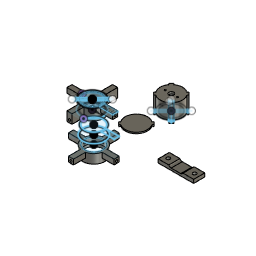
TurnstileAntenna (Autodesk Fusion 360 design; units mm, degrees)
Autodesk Fusion 360 part; units mm, degrees
note: some values were not read from the file. Set by a fixed rule: which face or edge a step refers to.
sketch "Sketch1" plane through (0, 0, 0) normal (0, 0, 1) x (1, 0, 0) in component "BOTTOM"
  circle A0 centre (0, 0) radius 20.15
  circle A1 centre (0, 0) radius 22
  dimension "d1" = 40.3
  constraint coincident A0.centre A1.centre
  measures "d1" diameter of A0
extrude "Extrude1" add sketch "Sketch1" along normal blind 17 and the other way blind 4 makes body 1 in component "BOTTOM"
sketch "Sketch1 (1)" plane through (0, 0, 17) normal (0, 0, 1) x (-1, 0, 0) in component "BOTTOM"
  circle A0 centre (0, 0) radius 20.15
  circle A1 centre (0, 0) radius 22
  circle A2 centre (0, 0) radius 20.15
  circle A3 centre (0, 0) radius 18
  point P0 (20.15, 0)
  constraint coincident A0.centre A1.centre
  constraint coincident A2 P0
extrude "Extrude2" add sketch "Sketch1 (1)" against normal blind 15 contours A0 A2 bodies 1 in component "BOTTOM"
sketch "Sketch2" plane through (0, 0, 17) normal (0, 0, 1) x (-1, 0, 0) in component "BOTTOM"
  line L0 (-20, 5) -> (-45, 5)
  line L1 (-45, 5) -> (-45, -5)
  line L2 (-45, -5) -> (-20, -5)
  line L3 (-20, -5) -> (-20, 5)
  dimension "d11" = 25
  dimension "d12" = 10
  constraint horizontal L0
  constraint vertical L1
  constraint horizontal L2
  constraint vertical L3
  measures "d11" distance of L0.start L0.end
  measures "d12" distance of L0.start L2.end
extrude "Extrude3" add sketch "Sketch2" along normal blind -9 and the other way blind 0 bodies 1 in component "BOTTOM"
pattern_circular "C-Pattern1" count 4 over 360 about axis through (0, 0, 1.75) along (0, 0, 1) of "Extrude3" in component "BOTTOM"
hole "Hole1" at (45, 0, 12.5) direction (-1, 0, 0) diameter 4.4 depth 99 tip angle 180 bodies 1 in component "BOTTOM"
extrude "Extrude4" add sketch "Sketch1 (1)" along normal blind -1 and the other way blind -1 contours A3 bodies 1 in component "BOTTOM"
extrude "Extrude5" add 1 faces at (1.6667, -29.2829, 17) along direction (0, 0, 1) blind 1 on bodies 1 bodies 1 in component "BOTTOM"
sketch "Sketch1 (2)" plane through (0, 0, 0) normal (0, 0, 1) x (1, 0, 0) in component "UPPER"
  circle A0 centre (0, 0) radius 20.1
  circle A1 centre (0, 0) radius 22
  dimension "d1_1" = 40.2
  constraint coincident A0.centre A1.centre
  measures "d1_1" diameter of A0
extrude "Extrude1'" add sketch "Sketch1 (2)" along normal blind 17 separate body makes body 2 in component "UPPER"
sketch "Sketch1 (1) (2)" plane through (0, 0, 17) normal (0, 0, 1) x (-1, 0, 0) in component "UPPER"
  circle A0 centre (0, 0) radius 20.1
  circle A1 centre (0, 0) radius 22
  circle A2 centre (0, 0) radius 20.1
  circle A3 centre (0, 0) radius 18
  point P0 (20.1, 0)
  constraint coincident A0.centre A1.centre
  constraint coincident A2 P0
extrude "Extrude2'" add sketch "Sketch1 (1) (2)" against normal blind 10 contours A0 A2 bodies 2 in component "UPPER"
sketch "Sketch2 (2)" plane through (0, 0, 17) normal (0, 0, 1) x (-1, 0, 0) in component "UPPER"
  line L0 (-20, 5) -> (-45, 5)
  line L1 (-45, 5) -> (-45, -5)
  line L2 (-45, -5) -> (-20, -5)
  line L3 (-20, -5) -> (-20, 5)
  dimension "d11_1" = 25
  dimension "d12_1" = 10
  constraint horizontal L0
  constraint vertical L1
  constraint horizontal L2
  constraint vertical L3
  measures "d11_1" distance of L0.start L0.end
  measures "d12_1" distance of L0.start L2.end
extrude "Extrude3'" add sketch "Sketch2 (2)" along normal blind -9 and the other way blind 0 bodies 2 in component "UPPER"
pattern_circular "C-Pattern1'" count 4 over 360 about axis through (0, 0, 1.75) along (0, 0, 1) of "Extrude3'" in component "UPPER"
hole "Hole1'" at (45, 0, 12.5) direction (-1, 0, 0) diameter 4.4 depth 99 tip angle 180 bodies 2 in component "UPPER"
hole "Hole2" at (0, -45, 12.5) direction (0, 1, 0) diameter 4.4 depth 99 tip angle 180 bodies 2 in component "UPPER"
extrude "Extrude4'" add sketch "Sketch1 (1) (2)" along normal blind -1 and the other way blind -1 contours A3 bodies 2 in component "UPPER"
extrude "Extrude5'" add 1 faces at (1.6667, -29.2829, 17) along direction (0, 0, 1) blind 1 on bodies 2 bodies 2 in component "UPPER"
sketch "Sketch3" plane through (0, 0, 18) normal (0, 0, 1) x (-1, 0, 0) in component "UPPER"
  arc A0 (-5, 21.4243) -> (-21.4243, 5) centre (0, 0) ccw
  line L0 (-21.4243, 5) -> (-45, 5)
  line L1 (-45, 5) -> (-45, -5)
  line L2 (-45, -5) -> (-21.4243, -5)
  arc A1 (-21.4243, -5) -> (-5, -21.4243) centre (0, 0) ccw
  line L3 (-5, -21.4243) -> (-5, -45)
  line L4 (-5, -45) -> (5, -45)
  line L5 (5, -45) -> (5, -21.4243)
  arc A2 (5, -21.4243) -> (21.4243, -5) centre (0, 0) ccw
  line L6 (21.4243, -5) -> (45, -5)
  line L7 (45, -5) -> (45, 5)
  line L8 (45, 5) -> (21.4243, 5)
  arc A3 (21.4243, 5) -> (5, 21.4243) centre (0, 0) ccw
  line L9 (5, 21.4243) -> (5, 45)
  line L10 (5, 45) -> (-5, 45)
  line L11 (-5, 45) -> (-5, 21.4243)
move_body "Move1" bodies 2 to x (1, 0, 0) y (0, 1, 0) z (0, 0, 1) at (0, 0, -35) in component "UPPER"
sketch "Sketch4" plane through (0, 0, -17) normal (0, 0, 1) x (-1, 0, 0) in component "UPPER"
  arc A0 (-5, 21.4243) -> (-21.4243, 5) centre (0, 0) ccw
  line L0 (-21.4243, 5) -> (-45, 5)
  line L1 (-45, 5) -> (-45, -5)
  line L2 (-45, -5) -> (-21.4243, -5)
  arc A1 (-21.4243, -5) -> (-5, -21.4243) centre (0, 0) ccw
  line L3 (-5, -21.4243) -> (-5, -45)
  line L4 (-5, -45) -> (5, -45)
  line L5 (5, -45) -> (5, -21.4243)
  arc A2 (5, -21.4243) -> (21.4243, -5) centre (0, 0) ccw
  line L6 (21.4243, -5) -> (45, -5)
  line L7 (45, -5) -> (45, 5)
  line L8 (45, 5) -> (21.4243, 5)
  arc A3 (21.4243, 5) -> (5, 21.4243) centre (0, 0) ccw
  line L9 (5, 21.4243) -> (5, 45)
  line L10 (5, 45) -> (-5, 45)
  line L11 (-5, 45) -> (-5, 21.4243)
  circle A4 centre (0, 0) radius 18
  constraint coincident A0.centre A1.centre
extrude "Extrude7" cut sketch "Sketch4" against normal blind 4 contours A4 bodies 2 in component "UPPER"
sketch "Sketch2 (3)" plane through (0, 0, 18) normal (0, 0, 1) x (-1, 0, 0) in component "CAP_UPPER"
  circle A0 centre (0, 0) radius 17.75
  circle A1 centre (0, 0) radius 22
  line L0 (-20, -20) -> (20, 20)
  line L1 (20, 15) -> (15, 20)
  line L2 (15, 20) -> (-20, -15)
  line L3 (-20, -15) -> (-15, -20)
  line L4 (-15, -20) -> (20, 15)
  line L5 (16, 16) -> (13.5, 18.5)
  line L6 (16, 16) -> (18.5, 13.5)
  line L7 (-16, -16) -> (-13.5, -18.5)
  line L8 (-16, -16) -> (-18.5, -13.5)
  line L9 (-13.1833, -18.1833) -> (-18.1833, -13.1833)
  line L10 (18.1898, 13.1898) -> (13.1898, 18.1898)
  dimension "d43" = 35.5
  dimension "d44" = 44
  constraint coincident A0.centre A1.centre
  constraint perpendicular L0 L1
  constraint perpendicular L1 L2
  constraint perpendicular L2 L3
  constraint perpendicular L1 L4
  constraint coincident L0 L5.start
  constraint coincident L2 L5.end
  constraint perpendicular L2 L5
  constraint coincident L4 L6.end
  constraint perpendicular L4 L6
  constraint coincident L0 L7.start
  constraint coincident L4 L7.end
  constraint perpendicular L4 L7
  constraint coincident L2 L8.end
  constraint perpendicular L2 L8
  constraint coincident L4 L9.start
  constraint coincident L2 L9.end
  constraint perpendicular L2 L9
  constraint coincident L4 L10.start
  constraint coincident L2 L10.end
  constraint perpendicular L2 L10
  measures "d43" diameter of A0
  measures "d44" diameter of A1
extrude "Extrude2''" add sketch "Sketch2 (3)" along normal blind 2.5 separate body contours A0 L4 | A0 A1 L4 | A0 L0 L4 | A0 A1 L0 L4 | A0 A1 L0 L4 | A0 L0 L2 | A0 A1 L0 L2 | A0 A1 L0 L2 | A0 L2 | A0 A1 L2 makes body 3 in component "CAP_UPPER"
extrude "Extrude3''" add sketch "Sketch2 (3)" against normal blind 1.5 contours A0 L4 | A0 L0 L4 | A0 L0 L2 | A0 L2 bodies 3 in component "CAP_UPPER"
sketch "Sketch4 (2)" plane through (0, 0, 18) normal (0, 0, 1) x (1, 0, 0) in component "BOTTOM"
  circle A0 centre (0, 0) radius 18
  constraint coincident A0.centre origin
sketch "Sketch5" plane through (0, 0, 0) normal (0, 0, 1) x (1, 0, 0) in component "BOTTOM"
  circle A0 centre (0, 0) radius 18
  dimension "d49" = 36
  constraint coincident A0.centre origin
  measures "d49" diameter of A0
extrude "Extrude8" cut sketch "Sketch5" along normal blind 58 bodies 1 in component "BOTTOM"
extrude "Extrude9" add 2 faces at (0, -37.3333, 8) (0, 37.3333, 8) along direction (0, 0, -1) blind 8 on bodies 1 bodies 1 in component "BOTTOM"
hole "Hole3" at (0, 45, 4.9894) direction (0, -1, 0) diameter 4.4 depth 99 tip angle 118 bodies 1 in component "BOTTOM"
extrude "Extrude4''" add sketch "Sketch2 (3)" along normal blind 2.5 contours A1 L0 L4 L10 | A1 L0 L4 L9 | A1 L0 L2 L10 | L0 L4 L6 L10 | A1 L0 L2 L9 | L0 L4 L7 L9 | L0 L2 L5 L10 | L0 L1 L4 L6 | L0 L2 L8 L9 | L0 L3 L4 L7 | L0 L1 L2 L5 | L0 L2 L3 L8 bodies 3 in component "CAP_UPPER"
extrude "Extrude5''" add sketch "Sketch2 (3)" against normal blind 1 contours L0 L4 L6 L10 | L0 L4 L7 L9 | L0 L2 L5 L10 | L0 L1 L4 L6 | L0 L2 L8 L9 | L0 L3 L4 L7 | L0 L1 L2 L5 | L0 L2 L3 L8 bodies 3 in component "CAP_UPPER"
sketch "Sketch2 (4)" plane through (0, 0, 18) normal (0, 0, 1) x (-1, 0, 0) in component "CAP_BOTTOM"
  circle A0 centre (0, 0) radius 17.75
  circle A1 centre (0, 0) radius 22
  line L0 (-20, -20) -> (20, 20)
  line L1 (20, 15) -> (15, 20)
  line L2 (15, 20) -> (-20, -15)
  line L3 (-20, -15) -> (-15, -20)
  line L4 (-15, -20) -> (20, 15)
  line L5 (16, 16) -> (13.5, 18.5)
  line L6 (16, 16) -> (18.5, 13.5)
  line L7 (-16, -16) -> (-13.5, -18.5)
  line L8 (-16, -16) -> (-18.5, -13.5)
  line L9 (-13.1833, -18.1833) -> (-18.1833, -13.1833)
  line L10 (18.1898, 13.1898) -> (13.1898, 18.1898)
  line L11 (0, 0) -> (-20, 20)
  line L12 (-20, 20) -> (20, -20)
  line L13 (15, -20) -> (20, -15)
  line L14 (20, -15) -> (-15, 20)
  line L15 (-15, 20) -> (-20, 15)
  line L16 (-20, 15) -> (15, -20)
  line L17 (16, -16) -> (13.5, -18.5)
  line L18 (16, -16) -> (18.5, -13.5)
  line L19 (18.1753, -13.1753) -> (13.1753, -18.1753)
  line L20 (-16, 16) -> (-18.5, 13.5)
  line L21 (-16, 16) -> (-13.5, 18.5)
  line L22 (-18.159, 13.159) -> (-13.159, 18.159)
  dimension "d43_1_1" = 35.5
  dimension "d44_1_1" = 44
  dimension "d65_1" = 3.5355
  constraint coincident A0.centre A1.centre
  constraint perpendicular L0 L1
  constraint perpendicular L1 L2
  constraint perpendicular L2 L3
  constraint perpendicular L1 L4
  constraint coincident L0 L5.start
  constraint coincident L2 L5.end
  constraint perpendicular L2 L5
  constraint coincident L4 L6.end
  constraint perpendicular L4 L6
  constraint coincident L0 L7.start
  constraint coincident L4 L7.end
  constraint perpendicular L4 L7
  constraint coincident L2 L8.end
  constraint perpendicular L2 L8
  constraint coincident L4 L9.start
  constraint coincident L2 L9.end
  constraint perpendicular L2 L9
  constraint coincident L4 L10.start
  constraint coincident L2 L10.end
  constraint perpendicular L2 L10
  constraint perpendicular L0 L11
  constraint perpendicular L0 L12
  constraint perpendicular L13 L14
  constraint perpendicular L14 L15
  constraint perpendicular L13 L16
  constraint coincident L12 L17.start
  constraint coincident L16 L17.end
  constraint perpendicular L16 L17
  constraint coincident L14 L19.start
  constraint coincident L16 L19.end
  constraint perpendicular L16 L19
  constraint coincident L11 L20.start
  constraint coincident L16 L20.end
  constraint perpendicular L16 L20
  constraint coincident L14 L21.end
  constraint perpendicular L14 L21
  constraint coincident L16 L22.start
  constraint coincident L14 L22.end
  constraint perpendicular L14 L22
  measures "d43_1_1" diameter of A0
  measures "d44_1_1" diameter of A1
  measures "d65_1" distance of L17.start L18.end
extrude "Extrude2'''" add sketch "Sketch2 (4)" along normal blind 2.5 separate body contours A0 L4 L14 | A0 A1 L4 L14 | A0 L0 L4 L14 | A0 A1 L0 L4 | A0 A1 L12 L14 | A0 L4 L12 L14 | A0 L0 L2 L14 | A0 A1 L0 L2 | L0 L4 L12 L14 | A0 A1 L12 L16 | A0 L4 L12 L16 | A0 L2 L14 | A0 A1 L2 L14 | L0 L2 L11 L12 L14 | L0 L4 L12 L16 | A0 A1 L4 L16 | A0 L4 L16 | A0 L2 L11 L12 L14 | A0 A1 L11 L12 L14 | L0 L2 L11 L12 L16 | A0 L0 L4 L16 | A0 A1 L0 L4 | A0 L2 L11 L12 L16 | A0 A1 L11 L12 L16 | A0 L0 L2 L16 | A0 A1 L0 L2 | A0 L2 L16 | A0 A1 L2 L16 makes body 4 in component "CAP_BOTTOM"
extrude "Extrude3'''" add sketch "Sketch2 (4)" against normal blind 1.5 contours A0 L4 L14 | A0 L0 L4 L14 | A0 L4 L12 L14 | A0 L0 L2 L14 | L0 L4 L12 L14 | A0 L4 L12 L16 | A0 L2 L14 | L0 L2 L11 L12 L14 | L0 L4 L12 L16 | A0 L4 L16 | A0 L2 L11 L12 L14 | L0 L2 L11 L12 L16 | A0 L0 L4 L16 | A0 L2 L11 L12 L16 | A0 L0 L2 L16 | A0 L2 L16 bodies 4 in component "CAP_BOTTOM"
extrude "Extrude4'''" add sketch "Sketch2 (4)" along normal blind 2.5 contours A1 L0 L4 L10 | A1 L12 L14 L19 | A1 L0 L2 L10 | L0 L4 L6 L10 | A1 L12 L16 L19 | L12 L14 L18 L19 | L0 L2 L5 L10 | L0 L1 L4 L6 | L12 L16 L17 L19 | L12 L13 L14 L18 | A1 L11 L12 L14 L22 | L0 L1 L2 L5 | A1 L0 L4 L9 | L12 L13 L16 L17 | A1 L11 L12 L16 L22 | L11 L12 L14 L21 L22 | A1 L0 L2 L9 | L0 L4 L7 L9 | L11 L12 L16 L20 L22 | L11 L12 L14 L15 L21 | L0 L2 L8 L9 | L0 L3 L4 L7 | L11 L12 L15 L16 L20 | L0 L2 L3 L8 bodies 4 in component "CAP_BOTTOM"
extrude "Extrude5'''" add sketch "Sketch2 (4)" against normal blind 4 contours L0 L4 L6 L10 | L12 L14 L18 L19 | L0 L2 L5 L10 | L0 L1 L4 L6 | L12 L16 L17 L19 | L12 L13 L14 L18 | L0 L1 L2 L5 | L12 L13 L16 L17 | L11 L12 L14 L21 L22 | L0 L4 L7 L9 | L11 L12 L16 L20 L22 | L11 L12 L14 L15 L21 | L0 L2 L8 L9 | L0 L3 L4 L7 | L11 L12 L15 L16 L20 | L0 L2 L3 L8 bodies 4 in component "CAP_BOTTOM"
extrude "Extrude6" cut 1 faces at (-2.6955, -3.38, 16.5) along direction (0, 0, 1) blind 2 on bodies 4 bodies 4 in component "CAP_BOTTOM"
sketch "Sketch3 (2)" plane through (0, 0, 0) normal (0, 0, 1) x (1, 0, 0) in component "CAP_BOTTOM"
  line L0 (0, -18) -> (-18, 0)
  line L1 (-17, -5) -> (-5, -17)
  circle A0 centre (0, 0) radius 17.55
  line L2 (-8.5019, -13.4981) -> (-9.6576, -14.6538)
  line L3 (-13.4868, -8.5132) -> (-14.6448, -9.6712)
  dimension "d66_1" = 35.1
  constraint coincident A0.centre origin
  constraint coincident L1 L2.start
  constraint coincident A0 L2.end
  constraint perpendicular L1 L2
  constraint coincident L1 L3.start
  constraint coincident A0 L3.end
  constraint perpendicular L1 L3
  measures "d66_1" diameter of A0
extrude "Extrude8'" cut sketch "Sketch3 (2)" along normal blind 26 bodies 4 in component "CAP_BOTTOM"
extrude "Extrude7'" add sketch "Sketch3 (2)" along normal blind 19 and the other way blind -14 contours L1 A0 L2 L3 bodies 4 in component "CAP_BOTTOM"
pattern_circular "C-Pattern1''" count 3 over 180 about axis through (0, 0, 1.75) along (0, 0, 1) both ways of "Extrude7'" in component "CAP_BOTTOM"
extrude "Extrude9'" add 3 faces at (-11.1761, -11.7447, 19) (-11.7447, 11.1761, 19) (11.7447, -11.1761, 19) along direction (0, 0, 1) blind 28.5 on bodies 4 bodies 4 in component "CAP_BOTTOM"
extrude "Extrude10" add 1 faces at (14.0867, -14.6401, 20.5) along direction (0, 0, 1) blind 27 on bodies 4 bodies 4 in component "CAP_BOTTOM"
sketch "Sketch4 (3)" plane through (0, 0, 47.5) normal (0, 0, 1) x (-1, 0, 0) in component "CAP_BOTTOM"
  arc A0 (-12.8542, -17.8542) -> (12.8542, -17.8542) centre (0, 0) ccw
  line L0 (12.8542, -17.8542) -> (15, -20)
  line L1 (15, -20) -> (20, -15)
  line L2 (20, -15) -> (17.8542, -12.8542)
  arc A1 (17.8542, -12.8542) -> (17.8542, 12.8542) centre (0, 0) ccw
  line L3 (17.8542, 12.8542) -> (20, 15)
  line L4 (20, 15) -> (15, 20)
  line L5 (15, 20) -> (12.8542, 17.8542)
  arc A2 (12.8542, 17.8542) -> (-12.8542, 17.8542) centre (0, 0) ccw
  line L6 (-12.8542, 17.8542) -> (-15, 20)
  line L7 (-15, 20) -> (-20, 15)
  line L8 (-20, 15) -> (-17.8542, 12.8542)
  arc A3 (-17.8542, 12.8542) -> (-17.8542, -12.8542) centre (0, 0) ccw
  line L9 (-17.8542, -12.8542) -> (-20, -15)
  line L10 (-20, -15) -> (-15, -20)
  line L11 (-15, -20) -> (-12.8542, -17.8542)
  arc A4 (9.6576, 14.6538) -> (-9.6712, 14.6448) centre (0, 0) ccw
  circle A5 centre (0, 0) radius 22.0311
  circle A6 centre (0, 0) radius 5
  line L12 (-13.4981, 8.5019) -> (-8.5132, 13.4868)
  line L13 (-8.5132, 13.4868) -> (-9.6712, 14.6448)
  line L14 (9.6576, 14.6538) -> (8.5019, 13.4981)
  line L15 (8.5019, 13.4981) -> (13.4868, 8.5132)
  line L16 (13.4868, 8.5132) -> (14.6448, 9.6712)
  arc A7 (14.6538, -9.6576) -> (14.6448, 9.6712) centre (0, 0) ccw
  line L17 (14.6538, -9.6576) -> (13.4981, -8.5019)
  line L18 (13.4981, -8.5019) -> (8.5132, -13.4868)
  line L19 (8.5132, -13.4868) -> (9.6712, -14.6448)
  arc A8 (-14.6538, 9.6576) -> (9.6712, -14.6448) centre (0, 0) ccw
  line L20 (-14.6538, 9.6576) -> (-13.4981, 8.5019)
  circle A9 centre (12, 0) radius 1.6
  circle A10 centre (-12, 0) radius 1.6
  dimension "d81" = 3.2
  dimension "d82" = 3.2
  constraint coincident A0.centre A1.centre
  constraint concentric A5 A6
  measures "d81" diameter of A9
  measures "d82" diameter of A10
extrude "Extrude11" add sketch "Sketch4 (3)" against normal blind 4 contours A4 L12 L13 L14 L15 L16 A7 L17 L18 L19 A8 L20 bodies 4 in component "CAP_BOTTOM"
sketch "Sketch1 (3)" plane through (0, 0, 0) normal (0, 0, 1) x (1, 0, 0) in component "BALCONY_HOLDER"
  circle A0 centre (165, -15) radius 3.5
  line L0 (165, -15) -> (217, -15)
  circle A1 centre (217, -15) radius 3.5
  line L1 (165, -15) -> (217, -15)
  line L2 (217, -15) -> (217, -4)
  line L3 (217, -4) -> (165, -4)
  line L4 (165, -4) -> (165, -15)
  line L5 (165, -15) -> (217, -15)
  line L6 (217, -15) -> (217, -26)
  line L7 (217, -26) -> (165, -26)
  line L8 (165, -26) -> (165, -15)
  line L9 (165, -4) -> (158, -4)
  line L10 (158, -4) -> (158, -15)
  line L11 (158, -15) -> (165, -15)
  line L12 (165, -15) -> (165, -4)
  line L13 (158, -15) -> (165, -15)
  line L14 (165, -15) -> (165, -26)
  line L15 (165, -26) -> (158, -26)
  line L16 (158, -26) -> (158, -15)
  line L17 (217, -15) -> (224, -15)
  line L18 (224, -15) -> (224, -4)
  line L19 (224, -4) -> (217, -4)
  line L20 (217, -4) -> (217, -15)
  line L21 (217, -15) -> (224, -15)
  line L22 (224, -15) -> (224, -26)
  line L23 (224, -26) -> (217, -26)
  line L24 (217, -26) -> (217, -15)
  line L25 (158, -4) -> (156, -4)
  line L26 (156, -4) -> (156, -26)
  line L27 (156, -26) -> (158, -26)
  line L28 (158, -26) -> (158, -4)
  line L29 (224, -4) -> (226, -4)
  line L30 (226, -4) -> (226, -26)
  line L31 (226, -26) -> (224, -26)
  line L32 (224, -26) -> (224, -4)
  line L33 (165, -15) -> (191, -15)
  line L34 (191, -15) -> (191, -26)
  line L35 (191, -26) -> (177, -26)
  line L36 (177, -26) -> (177, -3.8941)
  line L37 (177, -3.8941) -> (191, -3.8941)
  line L38 (191, -3.8941) -> (191, -26)
  line L39 (191, -3.8941) -> (205, -3.8941)
  line L40 (205, -3.8941) -> (205, -26)
  line L41 (205, -26) -> (191, -26)
  line L42 (191, -26) -> (191, -3.8941)
  dimension "d83" = 7
  dimension "d84" = 52
  dimension "d85" = 7
  dimension "d86" = 52
  dimension "d87" = 11
  dimension "d88" = 52
  dimension "d89" = 11
  dimension "d92" = 26
  dimension "d93" = 14
  dimension "d94" = 22.1059
  dimension "d95" = 14
  dimension "d96" = 22.1059
  constraint horizontal L0
  constraint coincident A0.centre L0.start
  constraint coincident L0.end A1.centre
  constraint horizontal L1
  constraint vertical L2
  constraint horizontal L3
  constraint vertical L4
  constraint horizontal L5
  constraint vertical L6
  constraint horizontal L7
  constraint vertical L8
  constraint horizontal L9
  constraint vertical L10
  constraint horizontal L11
  constraint vertical L12
  constraint horizontal L13
  constraint vertical L14
  constraint horizontal L15
  constraint vertical L16
  constraint horizontal L17
  constraint vertical L18
  constraint horizontal L19
  constraint vertical L20
  constraint horizontal L21
  constraint vertical L22
  constraint horizontal L23
  constraint vertical L24
  constraint horizontal L25
  constraint vertical L26
  constraint horizontal L27
  constraint vertical L28
  constraint horizontal L29
  constraint vertical L30
  constraint horizontal L31
  constraint vertical L32
  constraint horizontal L33
  constraint midpoint L7 L34.end
  constraint horizontal L35
  constraint vertical L36
  constraint horizontal L37
  constraint vertical L38
  constraint horizontal L39
  constraint vertical L40
  constraint horizontal L41
  constraint vertical L42
  measures "d83" diameter of A0
  measures "d84" distance of A0.centre L0.end
  measures "d85" diameter of A1
  measures "d86" distance of A0.centre L0.end
  measures "d87" distance of A0.centre L3.end
  measures "d88" distance of A0.centre L0.end
  measures "d89" distance of A0.centre L7.end
  measures "d92" distance of A0.centre L33.end
  measures "d93" distance of L34.end L35.end
  measures "d94" distance of L34.end L37.end
  measures "d95" distance of L37.end L39.end
  measures "d96" distance of L37.end L34.end
extrude "Extrude1''" add sketch "Sketch1 (3)" along normal blind 7 separate body contours A0 L0 L1 L5 L7 L8 L14 L33 L36 | A0 L0 L1 L3 L4 L5 L12 L33 L36 | A0 L4 L9 L10 L11 L12 L13 L28 | A0 L8 L11 L13 L14 L15 L16 L28 | L0 L1 L3 L5 L33 L36 L38 L42 | L0 L1 L5 L7 L33 L34 L35 L36 L38 L42 | L0 L1 L3 L5 L38 L40 L42 | L0 L1 L5 L7 L34 L38 L40 L41 L42 | L10 L16 L25 L26 L27 L28 | L0 A1 L1 L2 L3 L5 L20 L40 | L0 A1 L1 L5 L6 L7 L24 L40 | A1 L2 L17 L18 L19 L20 L21 L32 | A1 L6 L17 L21 L22 L23 L24 L32 | L18 L22 L29 L30 L31 L32 makes body 5 in component "BALCONY_HOLDER"
sketch "Sketch2 (5)" plane through (0, 0, 7) normal (0, 0, 1) x (-1, 0, 0) in component "BALCONY_HOLDER"
  circle A0 centre (-217, 15) radius 3.5
  circle A1 centre (-165, 15) radius 3.5
  line L0 (-226, 4) -> (-156, 4)
  line L1 (-156, 4) -> (-156, 26)
  line L2 (-156, 26) -> (-226, 26)
  line L3 (-226, 26) -> (-226, 4)
  line L4 (-165, 15) -> (-191, 15) construction
  line L5 (-191, 15) -> (-191, 26) construction
  line L6 (-191, 26) -> (-177, 26)
  line L7 (-177, 26) -> (-177, 4)
  line L8 (-177, 4) -> (-191, 4)
  line L9 (-191, 4) -> (-191, 26)
  line L10 (-191, 26) -> (-205, 26)
  line L11 (-205, 26) -> (-205, 4)
  line L12 (-205, 4) -> (-191, 4)
  line L13 (-191, 4) -> (-191, 26)
  dimension "d97" = 26
  dimension "d98" = 14
  dimension "d99" = 22
  dimension "d100" = 14
  dimension "d101" = 22
  constraint coincident A1.centre L4.start
  constraint horizontal L4
  constraint midpoint L2 L5.end
  constraint horizontal L6
  constraint vertical L7
  constraint horizontal L8
  constraint vertical L9
  constraint horizontal L10
  constraint vertical L11
  constraint horizontal L12
  constraint vertical L13
  measures "d97" distance of A1.centre L4.end
  measures "d98" distance of L5.end L6.end
  measures "d99" distance of L5.end L8.end
  measures "d100" distance of L5.end L10.end
  measures "d101" distance of L5.end L8.end
extrude "Extrude2''''" cut sketch "Sketch2 (5)" against normal blind 3 contours L0 L2 L9 L10 L11 L12 L13 | L0 L2 L6 L7 L8 L9 L13 bodies 5 in component "BALCONY_HOLDER"
fillet "Fillet1" radius 5 2 edges at (205, -15, 4) (177, -15, 4) on bodies 5 in component "BALCONY_HOLDER"
move_body "Move1'" bodies 3 to x (1, 0, 0) y (0, 1, 0) z (0, 0, 1) at (87, 0, 0) in component "CAP_UPPER"
component "BOTTOM" placed x (1, 0, 0) y (0, 1, 0) z (0, 0, 1) at (0, 0, 0)
component "UPPER" placed x (1, 0, 0) y (0, 1, 0) z (0, 0, 1) at (78, -75, 34)
component "CAP_UPPER" placed x (1, 0, 0) y (0, 1, 0) z (0, 0, 1) at (0, 0, 0)
component "CAP_BOTTOM" placed x (1, 0, 0) y (0, 1, 0) z (0, 0, 1) at (98, 58, 0)
component "BALCONY_HOLDER" placed x (1, 0, 0) y (0, 1, 0) z (0, 0, 1) at (0, 0, 0)
